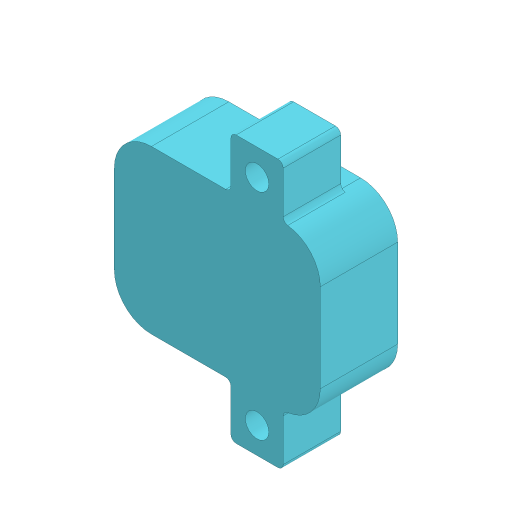
# Autodesk Inventor part: PrzyciskSTOP_1
Saved by Autodesk Inventor 2024.3 (Build 283343000, 343)
## iProperties
Created: 2025-08-19
Part Number: PrzyciskSTOP_1
Material: Generic
Document SubType Name: Modeling
Designer: PM
Density: 1 g/cm^3
Appearance: Cadet Blue
Author: PM
## iProperties of the stored document PrzyciskSTOP_1_3DPrint.ipt
Created: 2025-08-19
Part Number: PrzyciskSTOP_1_3DPrint
Material: Generic
Document SubType Name: Modeling
Designer: PM
Density: 1 g/cm^3
Appearance: Default
Author: PM
Autodesk Inventor part; units mm, degrees
ref_plane "YZ Plane" through (0, 0, 0) normal (1, 0, 0) x (0, 1, 0)
ref_plane "XZ Plane" through (0, 0, 0) normal (0, 1, 0) x (-1, 0, 0)
ref_plane "XY Plane" through (0, 0, 0) normal (0, 0, 1) x (1, 0, 0)
sketch "Sketch1" plane through (0, 0, 0) normal (0, 0, 1) x (1, 0, 0)
  arc A0 (-12.6, 10.95) -> (-15.1, 8.45) centre (-12.6, 8.45) ccw projected
  line L0 (-15.1, 8.45) -> (-15.1, -8.45) projected
  arc A1 (-15.1, -8.45) -> (-12.6, -10.95) centre (-12.6, -8.45) ccw projected
  line L1 (-12.6, -10.95) -> (12.6, -10.95) projected
  arc A2 (12.6, -10.95) -> (15.1, -8.45) centre (12.6, -8.45) ccw projected
  line L2 (15.1, -8.45) -> (15.1, 8.45) projected
  arc A3 (15.1, 8.45) -> (12.6, 10.95) centre (12.6, 8.45) ccw projected
  line L3 (12.6, 10.95) -> (-12.6, 10.95) projected
  circle A4 centre (11.825, 7.675) radius 1.575 projected
  circle A5 centre (11.825, -7.675) radius 1.575 projected
  line L4 (15.7, 8.45) -> (15.7, -8.45)
  arc A6 (12.6, -11.55) -> (15.7, -8.45) centre (12.6, -8.45) ccw
  line L5 (12.6, -11.55) -> (-12.6, -11.55)
  arc A7 (-15.7, -8.45) -> (-12.6, -11.55) centre (-12.6, -8.45) ccw
  line L6 (-15.7, -8.45) -> (-15.7, 8.45)
  arc A8 (-12.6, 11.55) -> (-15.7, 8.45) centre (-12.6, 8.45) ccw
  line L7 (-12.6, 11.55) -> (12.6, 11.55)
  arc A9 (15.7, 8.45) -> (12.6, 11.55) centre (12.6, 8.45) ccw
  line L8 (19.7, -8.45) -> (19.7, 8.45)
  arc A10 (19.7, 8.45) -> (12.6, 15.55) centre (12.6, 8.45) ccw
  line L9 (12.6, 15.55) -> (-12.6, 15.55)
  arc A11 (-12.6, 15.55) -> (-19.7, 8.45) centre (-12.6, 8.45) ccw
  line L10 (-19.7, 8.45) -> (-19.7, -8.45)
  arc A12 (-19.7, -8.45) -> (-12.6, -15.55) centre (-12.6, -8.45) ccw
  line L11 (-12.6, -15.55) -> (12.6, -15.55)
  arc A13 (12.6, -15.55) -> (19.7, -8.45) centre (12.6, -8.45) ccw
  point P0 (0, 0)
  dimension "d0" = 0.6
  dimension "d1" = 4
  constraints: 16 end point, 16 point on circle, 8 centre point, 14 other
  measures "d0" distance between parallel lines of L2 L4
  measures "d1" distance between parallel lines of L4 L8
extrude "Extrusion1" add sketch "Sketch1" along normal blind 5 contours L3 A3 L2 A2 L1 A1 L0 A0 | A4 | A5 | L4 A6 L5 A7 L6 A8 L7 A9 | A13 L11 A12 L10 A11 L9 A10 L8
sketch "Sketch2" plane through (0, 0, 0) normal (0, 0, -1) x (-1, 0, 0)
  line L0 (12.6, 11.55) -> (-12.6, 11.55) projected
  arc A0 (15.7, 8.45) -> (12.6, 11.55) centre (12.6, 8.45) ccw projected
  line L1 (15.7, -8.45) -> (15.7, 8.45) projected
  arc A1 (12.6, -11.55) -> (15.7, -8.45) centre (12.6, -8.45) ccw projected
  line L2 (12.6, -10.95) -> (-12.6, -10.95) projected
  arc A2 (-15.7, -8.45) -> (-12.6, -11.55) centre (-12.6, -8.45) ccw projected
  line L3 (-15.7, 8.45) -> (-15.7, -8.45) projected
  arc A3 (-12.6, 11.55) -> (-15.7, 8.45) centre (-12.6, 8.45) ccw projected
  arc A4 (-12.6, 15.55) -> (-19.7, 8.45) centre (-12.6, 8.45) ccw projected
  line L4 (-19.7, -8.45) -> (-19.7, 8.45) projected
  arc A5 (-19.7, -8.45) -> (-12.6, -15.55) centre (-12.6, -8.45) ccw projected
  line L5 (12.6, -15.55) -> (-12.6, -15.55) projected
  arc A6 (12.6, -15.55) -> (19.7, -8.45) centre (12.6, -8.45) ccw projected
  line L6 (19.7, 8.45) -> (19.7, -8.45) projected
  arc A7 (19.7, 8.45) -> (12.6, 15.55) centre (12.6, 8.45) ccw projected
  line L7 (-12.6, 15.55) -> (12.6, 15.55) projected
  line L8 (7.1, -5) -> (15.1, -5) projected
  line L9 (15.1, -5) -> (15.1, 5) projected
  line L10 (15.1, 5) -> (7.1, 5) projected
  line L11 (7.1, 5) -> (7.1, -5) projected
  line L12 (15.7, 7) -> (19.7, 7)
  line L13 (19.7, 7) -> (19.7, -7)
  line L14 (19.7, -7) -> (15.7, -7)
  line L15 (15.7, -7) -> (15.7, 7)
  line L16 (15.7, 7) -> (19.7, -7) construction
  line L17 (19.7, 7) -> (15.7, -7) construction
  line L18 (-12.6, -11.55) -> (12.6, -11.55) projected
  point P0 (0, 0)
  point P1 (17.7, 0)
  point P2 (19.7, 0)
  point P3 (17.7, 7)
  dimension "d4" = 2
  constraints: 12 end point, 4 midpoint, 2 parallel, 2 point on line, 1 horizontal, 1 horizontal alignment, 1 perpendicular
  measures "d4" distance from line of L10 point (17.7, 7)
extrude "Extrusion2" add sketch "Sketch2" along normal blind 9.8 contours L0 A3 L3 A2 L18 A1 L1 L14 L6 A6 L5 A5 L4 A4 L7 A7 L12 A0
sketch "Sketch3" plane through (0, 0, 0) normal (0, 0, -1) x (-1, 0, 0)
  circle A0 centre (-11.825, -7.675) radius 1.575 projected
  circle A1 centre (-11.825, 7.675) radius 1.575 projected
  circle A2 centre (-11.825, -7.675) radius 1.2
  circle A3 centre (-11.825, 7.675) radius 1.2
  point P0 (0, 0)
  dimension "d7" = 3.15
  dimension "d8" = 2.4
  dimension "d9" = 2.4
  constraints: 2 centre point, 2 coincident
  measures "d7" diameter of A0
  measures "d8" diameter of A2
  measures "d9" diameter of A3
extrude "Extrusion3" cut sketch "Sketch3" against normal blind 3 contours A2 | A3
sketch "Sketch4" plane through (0, 0, 5) normal (0, 0, 1) x (1, 0, 0)
  arc A0 (19.7, 8.45) -> (12.6, 15.55) centre (12.6, 8.45) ccw projected
  line L0 (12.6, 15.55) -> (-12.6, 15.55) projected
  arc A1 (-12.6, 15.55) -> (-19.7, 8.45) centre (-12.6, 8.45) ccw projected
  line L1 (-19.7, 8.45) -> (-19.7, -8.45) projected
  arc A2 (-19.7, -8.45) -> (-12.6, -15.55) centre (-12.6, -8.45) ccw projected
  line L2 (-12.6, -15.55) -> (12.6, -15.55) projected
  arc A3 (12.6, -15.55) -> (19.7, -8.45) centre (12.6, -8.45) ccw projected
  line L3 (19.7, -8.45) -> (19.7, 8.45) projected
  line L4 (-2.6, -15.55) -> (-12.6, -15.55)
  line L5 (-12.6, -15.55) -> (-12.6, -25.55)
  line L6 (-12.6, -25.55) -> (-2.6, -25.55)
  line L7 (-2.6, -25.55) -> (-2.6, -15.55)
  line L8 (-2.6, -15.55) -> (-12.6, -25.55) construction
  line L9 (-12.6, -15.55) -> (-2.6, -25.55) construction
  line L10 (-12.6, -15.55) -> (12.6, -15.55) projected
  line L11 (19.7, 0) -> (-19.7, 0)
  line L12 (0, 15.55) -> (0, -15.55)
  line L13 (-2.6, 15.55) -> (-12.6, 15.55)
  line L14 (-12.6, 15.55) -> (-12.6, 25.55)
  line L15 (-12.6, 25.55) -> (-2.6, 25.55)
  line L16 (-2.6, 25.55) -> (-2.6, 15.55)
  line L17 (-2.6, 15.55) -> (-12.6, 25.55) construction
  line L18 (-12.6, 15.55) -> (-2.6, 25.55) construction
  arc A4 (19.7, 8.45) -> (12.6, 15.55) centre (12.6, 8.45) ccw
  line L19 (2.6, 15.55) -> (12.6, 15.55)
  line L20 (2.6, 25.55) -> (2.6, 15.55)
  line L21 (2.6, 15.55) -> (12.6, 25.55) construction
  line L22 (12.6, 25.55) -> (2.6, 25.55)
  line L23 (12.6, 15.55) -> (2.6, 25.55) construction
  line L24 (12.6, 15.55) -> (12.6, 25.55)
  line L25 (2.6, -15.55) -> (12.6, -15.55)
  line L26 (2.6, -25.55) -> (2.6, -15.55)
  line L27 (2.6, -15.55) -> (12.6, -25.55) construction
  line L28 (12.6, -15.55) -> (2.6, -25.55) construction
  line L29 (12.6, -15.55) -> (12.6, -25.55)
  line L30 (12.6, -25.55) -> (2.6, -25.55)
  point P0 (0, 0)
  point P1 (-7.6, -20.55)
  point P2 (-7.6, 20.55)
  point P3 (7.6, 20.55)
  point P4 (2.6, 15.55)
  point P5 (-2.6, 15.55)
  point P6 (7.6, -20.55)
  point P7 (2.6, -15.55)
  dimension "d12" = 10
  dimension "d13" = 10
  constraints: 52 end point, 13 symmetric about line, 6 midpoint, 2 parallel, 2 point on circle, 1 centre point, 1 horizontal, 1 perpendicular, 1 other
  measures "d12" distance of L2.start L5.end
  measures "d13" distance of L5.end L6.end
extrude "Extrusion4" add sketch "Sketch4" against normal blind 11 contours L0 L20 L22 L24 | L29 L30 L26 L2
sketch "Sketch5" plane through (0, 0, -6) normal (0, 0, -1) x (-1, 0, 0)
  line L0 (-12.6, -15.55) -> (-2.6, -15.55) projected
  line L1 (5.6, -22.55) -> (12.6, -15.55)
  line L2 (4.1, -17.05) -> (11.1, -24.05)
  line L3 (12.6, -11.55) -> (-12.6, -11.55) projected
  arc A0 (-15.7, -8.45) -> (-12.6, -11.55) centre (-12.6, -8.45) ccw projected
  line L4 (-15.7, -8.45) -> (-15.7, 8.45) projected
  arc A1 (-12.6, 11.55) -> (-15.7, 8.45) centre (-12.6, 8.45) ccw projected
  line L5 (-12.6, 11.55) -> (12.6, 11.55) projected
  arc A2 (15.7, 8.45) -> (12.6, 11.55) centre (12.6, 8.45) ccw projected
  line L6 (15.7, 8.45) -> (15.7, 7) projected
  line L7 (15.7, 7) -> (19.7, 7) projected
  line L8 (19.7, 7) -> (19.7, 8.45) projected
  arc A3 (19.7, 8.45) -> (12.6, 15.55) centre (12.6, 8.45) ccw projected
  line L9 (12.6, 15.55) -> (-12.6, 15.55) projected
  arc A4 (-12.6, 15.55) -> (-19.7, 8.45) centre (-12.6, 8.45) ccw projected
  line L10 (-19.7, 8.45) -> (-19.7, -8.45) projected
  arc A5 (-19.7, -8.45) -> (-12.6, -15.55) centre (-12.6, -8.45) ccw projected
  line L11 (-12.6, -15.55) -> (12.6, -15.55) projected
  arc A6 (12.6, -15.55) -> (19.7, -8.45) centre (12.6, -8.45) ccw projected
  line L12 (19.7, -8.45) -> (19.7, -7) projected
  line L13 (19.7, -7) -> (15.7, -7) projected
  line L14 (15.7, -7) -> (15.7, -8.45) projected
  arc A7 (12.6, -11.55) -> (15.7, -8.45) centre (12.6, -8.45) ccw projected
  circle A8 centre (-11.825, 7.675) radius 1.2 projected
  circle A9 centre (-11.825, -7.675) radius 1.2 projected
  line L15 (19.7, 7) -> (15.7, 7) projected
  line L16 (15.7, 7) -> (15.7, 8.45) projected
  arc A10 (15.7, 8.45) -> (12.6, 11.55) centre (12.6, 8.45) ccw projected
  line L17 (12.6, 11.55) -> (-12.6, 11.55) projected
  arc A11 (-12.6, 11.55) -> (-15.7, 8.45) centre (-12.6, 8.45) ccw projected
  line L18 (-15.7, 8.45) -> (-15.7, -8.45) projected
  arc A12 (-15.7, -8.45) -> (-12.6, -11.55) centre (-12.6, -8.45) ccw projected
  line L19 (-12.6, -11.55) -> (12.6, -11.55) projected
  arc A13 (12.6, -11.55) -> (15.7, -8.45) centre (12.6, -8.45) ccw projected
  line L20 (15.7, -8.45) -> (15.7, -7) projected
  line L21 (15.7, -7) -> (19.7, -7) projected
  line L22 (19.7, 7) -> (19.7, -7) projected
  line L23 (19.7, 0) -> (-19.7, 0)
  line L24 (0, -15.55) -> (0, 15.55)
  line L25 (-12.6, -15.55) -> (-12.6, -25.55) projected
  line L26 (-12.6, -25.55) -> (-2.6, -25.55) projected
  line L27 (-2.6, -25.55) -> (-2.6, -15.55) projected
  point P0 (0, 0)
  point P1 (7.6, -20.55)
  point P2 (7.6, 20.55)
  point P3 (-7.6, 20.55)
  point P4 (-7.6, -20.55)
  constraints: 8 end point, 5 midpoint, 3 symmetric about line, 1 perpendicular
hole "Hole1" at (7.6, 20.55, -6) at (7.6, -20.55, -6) direction (0, 0, 1) diameter 4.5 end through all clearance for "Countersunk Flat Head Hex Socket Screw ISO 10642" size "M4" standard "ISO"
fillet "Fillet1" radius 1 2 edges at (12.6, -15.55, -0.5) (12.6, 15.55, -0.5)
fillet "Fillet2" radius 1 6 edges at (2.6, -15.55, -0.5) (2.6, 15.55, -0.5) (12.6, 25.55, -0.5) (2.6, 25.55, -0.5) (2.6, -25.55, -0.5) (12.6, -25.55, -0.5)
sketch "Sketch6" plane through (0, 0, -9.8) normal (0, 0, -1) x (-1, 0, 0)
  line L0 (12.6, -11.55) -> (-12.6, -11.55) projected
  arc A0 (-15.7, -8.45) -> (-12.6, -11.55) centre (-12.6, -8.45) ccw projected
  line L1 (-15.7, -8.45) -> (-15.7, 8.45) projected
  arc A1 (-12.6, 11.55) -> (-15.7, 8.45) centre (-12.6, 8.45) ccw projected
  line L2 (-12.6, 11.55) -> (12.6, 11.55) projected
  arc A2 (15.7, 8.45) -> (12.6, 11.55) centre (12.6, 8.45) ccw projected
  line L3 (15.7, 8.45) -> (15.7, 7) projected
  line L4 (15.7, 7) -> (19.7, 7) projected
  line L5 (19.7, 7) -> (19.7, 8.45) projected
  arc A3 (19.7, 8.45) -> (12.6, 15.55) centre (12.6, 8.45) ccw projected
  line L6 (12.6, 15.55) -> (-13.2535, 15.55) projected
  arc A4 (-13.4765, 15.4957) -> (-13.2535, 15.55) centre (-13.6, 16.488) ccw projected
  arc A5 (-13.4765, 15.4957) -> (-19.7, 8.45) centre (-12.6, 8.45) ccw projected
  line L7 (-19.7, 8.45) -> (-19.7, -8.45) projected
  arc A6 (-19.7, -8.45) -> (-13.4765, -15.4957) centre (-12.6, -8.45) ccw projected
  arc A7 (-13.2535, -15.55) -> (-13.4765, -15.4957) centre (-13.6, -16.488) ccw projected
  line L8 (-13.2535, -15.55) -> (12.6, -15.55) projected
  arc A8 (12.6, -15.55) -> (19.7, -8.45) centre (12.6, -8.45) ccw projected
  line L9 (19.7, -8.45) -> (19.7, -7) projected
  line L10 (19.7, -7) -> (15.7, -7) projected
  line L11 (15.7, -7) -> (15.7, -8.45) projected
  arc A9 (12.6, -11.55) -> (15.7, -8.45) centre (12.6, -8.45) ccw projected
  arc A10 (-12.6, 15.55) -> (-19.7, 8.45) centre (-12.6, 8.45) ccw projected
  arc A11 (-19.7, -8.45) -> (-12.6, -15.55) centre (-12.6, -8.45) ccw projected
  point P0 (0, 0)
extrude "Extrusion5" cut sketch "Sketch6" against normal up to surface (3.8 mm away) contours L8 A7 A11 | A4 L6 A10
equation "\"d9\" = d8"
body "Solid1"
